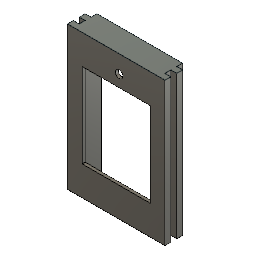
SOPORTE TECLADO v3 (Autodesk Fusion 360 design; units mm, degrees)
Autodesk Fusion 360 part; units mm, degrees
sketch "Boceto1" plane through (0, 0, 0) normal (0, 0, 1) x (1, 0, 0)
  line L0 (0, 0) -> (46, 0)
  line L1 (46, 0) -> (46, 57)
  line L2 (46, 57) -> (0, 57)
  line L3 (0, 57) -> (0, 0)
  line L4 (-6, 77) -> (52, 77)
  line L5 (52, 77) -> (52, -20)
  line L6 (52, -20) -> (-6, -20)
  line L7 (-6, -20) -> (-6, 77)
  dimension "d1" = 46
  dimension "d2" = 57
  dimension "d3" = 58
  dimension "d4" = 97
  dimension "d5" = 6
  dimension "d6" = 20
  constraint horizontal L0
  constraint vertical L1
  constraint horizontal L2
  constraint vertical L3
  constraint coincident L0.start L3.end
  constraint horizontal L4
  constraint vertical L5
  constraint horizontal L6
  constraint vertical L7
  measures "d1" distance of L0.start L0.end
  measures "d2" distance of L0.start L2.end
  measures "d3" distance of L4.start L4.end
  measures "d4" distance of L4.start L6.end
  measures "d5" distance of L1 L5
  measures "d6" distance of L0 L6
extrude "Extruir1" add sketch "Boceto1" against normal blind 2
sketch "Boceto2" plane through (0, 0, -2) normal (0, 0, -1) x (-1, 0, 0)
  line L0 (0, 57) -> (0, 0)
  line L1 (0, 0) -> (-46, 0)
  line L2 (-46, 0) -> (-46, 57)
  line L3 (-46, 57) -> (0, 57)
  line L4 (-52, -20) -> (6, -20)
  line L5 (6, -20) -> (6, 77)
  line L6 (6, 77) -> (-52, 77)
  line L7 (-52, 77) -> (-52, -20)
  line L8 (-46, 57) -> (0, 57)
  line L9 (0, 57) -> (0, 0)
  line L10 (0, 0) -> (-46, 0)
  line L11 (-46, 0) -> (-46, 57)
  line L12 (-49, -17) -> (3, -17)
  line L13 (3, -17) -> (3, 74)
  line L14 (3, 74) -> (-49, 74)
  line L15 (-49, 74) -> (-49, -17)
  circle A0 centre (-25, 65) radius 2.5
  dimension "d9" = -3
  dimension "d10" = 5
  constraint horizontal L8
  constraint vertical L9
  constraint horizontal L10
  constraint vertical L11
  constraint coincident L0.end L1.start
  constraint coincident L2.end L3.start
  measures "d10" diameter of A0
extrude "Extruir2" add sketch "Boceto2" along normal blind 14 contours L4 L5 L6 L7
sketch "Boceto3" plane through (0, -17, 0) normal (0, 1, 0) x (-1, 0, 0)
  line L0 (3, -2) -> (-49, -2)
  line L1 (-49, -2) -> (-49, -16)
  line L2 (-49, -16) -> (3, -16)
  line L3 (3, -16) -> (3, -2)
  line L4 (-23, -9) -> (-31, -9)
  ellipse E0 centre (-23, -9) end of major axis (-31, -9) minor radius 4
  line L5 (-15, -9) -> (-31, -9)
  line L6 (-23, -5) -> (-23, -13)
  dimension "d14" = 8
  constraint horizontal L4
  constraint coincident E0 L5.start
  constraint coincident L4.end E0
  constraint coincident E0 L6.start
  constraint coincident E0 L6.end
  measures "d14" distance of L4.start L4.end
extrude "Extruir3" cut sketch "Boceto3" against normal blind 10 contours L4 E0 L5 L6 | E0 L5 L6 | L4 E0 L5 L6 | E0 L5 L6
extrude "Extruir4" cut sketch "Boceto2" against normal blind 10 contours A0
sketch "Boceto4" plane through (0, 77, 0) normal (0, 1, 0) x (-1, 0, 0)
  line L0 (6, 0) -> (-52, 0)
  line L1 (-52, 0) -> (-52, -16)
  line L2 (-52, -16) -> (6, -16)
  line L3 (6, -16) -> (6, 0)
  line L4 (-52, 0) -> (-52, -16)
  line L5 (-52, 0) -> (-56, 0)
  line L6 (-56, 0) -> (-52, 0)
  line L7 (-52, 0) -> (-52, -4)
  line L8 (-52, -4) -> (-56, -4)
  line L9 (-56, -4) -> (-56, 0)
  line L10 (-52, -4) -> (-52, -8)
  line L11 (-52, -8) -> (-56, -8)
  line L12 (-56, -8) -> (-56, -12)
  line L13 (-56, -12) -> (-52, -12)
  line L14 (-52, -12) -> (-52, -8)
  line L15 (-23, 0) -> (-23, -16)
  line L16 (6, -4) -> (10, -4)
  line L17 (6, 0) -> (10, 0)
  line L18 (10, -4) -> (10, 0)
  line L19 (6, -8) -> (10, -8)
  line L20 (10, -8) -> (10, -12)
  line L21 (10, -12) -> (6, -12)
  dimension "d19" = 4
  dimension "d20" = 4
  dimension "d21" = 4
  dimension "d22" = 4
  dimension "d23" = 4
  dimension "d24" = 4
  constraint coincident L0.end L1.start
  constraint coincident L1.end L2.start
  constraint perpendicular L4 L5
  constraint horizontal L6
  constraint vertical L7
  constraint horizontal L8
  constraint vertical L9
  constraint midpoint L1 L10.end
  constraint horizontal L11
  constraint vertical L12
  constraint horizontal L13
  constraint vertical L14
  constraint midpoint L0 L15.start
  constraint perpendicular L0 L15
  constraint symmetric L0.end L15 L0.start
  constraint symmetric L5.end L15 L17.end
  constraint symmetric L7.end L15 L16.start
  constraint symmetric L8.end L15 L16.end
  constraint symmetric L10.end L15 L19.start
  constraint symmetric L11.end L15 L19.end
  constraint symmetric L12.end L15 L20.end
  constraint symmetric L13.end L15 L21.end
  measures "d19" distance of L0.end L5.end
  measures "d20" distance of L5.end L0.end
  measures "d21" distance of L5.end L8.end
  measures "d22" distance of L7.end L10.end
  measures "d23" distance of L10.end L11.end
  measures "d24" distance of L10.end L13.end
extrude "Extruir5" add sketch "Boceto4" against normal blind 97 contours L3 L16 L17 L18 | L1 L4 L5 L6 L7 L8 L9 | L3 L19 L20 L21 | L1 L4 L11 L12 L13 L14
sketch "Boceto5" plane through (0, 77, 0) normal (0, 1, 0) x (-1, 0, 0)
  line L0 (10, 0) -> (-56, 0)
  line L1 (-56, 0) -> (-56, -4)
  line L2 (-56, -4) -> (-52, -4)
  line L3 (-52, -4) -> (-52, -8)
  line L4 (-52, -8) -> (-56, -8)
  line L5 (-56, -8) -> (-56, -12)
  line L6 (-56, -12) -> (-52, -12)
  line L7 (-52, -12) -> (-52, -16)
  line L8 (-52, -16) -> (6, -16)
  line L9 (6, -16) -> (6, -12)
  line L10 (6, -12) -> (10, -12)
  line L11 (10, -12) -> (10, -8)
  line L12 (10, -8) -> (6, -8)
  line L13 (6, -8) -> (6, -4)
  line L14 (6, -4) -> (10, -4)
  line L15 (10, -4) -> (10, 0)
